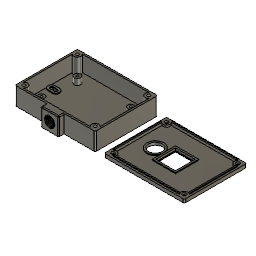
ESP32-FridgeStat Case (Autodesk Fusion 360 design; units mm, degrees)
part number: 2026-06-30-17-07-55-763
Autodesk Fusion 360 part; units mm, degrees
note: some values were not read from the file. Chosen so that the rebuilt part matches the saved one: which bodies a step acts on; which face or edge a step refers to; how an offset face is resized. Set by a fixed rule: which sketch regions a step uses.
sketch "Sketch1" plane through (0, 0, 0) normal (0, 0, 1) x (1, 0, 0)
  line L0 (0, 0) -> (90, 0)
  line L1 (90, 0) -> (90, 70)
  line L2 (90, 70) -> (0, 70)
  line L3 (0, 70) -> (0, 0)
  line L4 (99.999, 69.9991) -> (189.999, 69.9991)
  line L5 (189.999, 69.9991) -> (189.999, -0.0009)
  line L6 (189.999, -0.0009) -> (99.999, -0.0009)
  line L7 (99.999, -0.0009) -> (99.999, 69.9991)
  dimension "d1" = 90
  dimension "d2" = 70
  dimension "d126" = 90
  dimension "d127" = 70
  constraint horizontal L0
  constraint vertical L1
  constraint horizontal L2
  constraint vertical L3
  constraint coincident L0.start L3.end
  constraint horizontal L4
  constraint vertical L5
  constraint horizontal L6
  constraint vertical L7
  measures "d1" distance of L0.start L0.end
  measures "d2" distance of L0.start L2.end
  measures "d126" distance of L4.start L4.end
  measures "d127" distance of L4.start L6.end
extrude "Extrude1" add sketch "Sketch1" along normal blind 2 makes body 1 at (30, 46.6667, 0) makes body 2 at (129.999, 46.6657, 0)
sketch "Sketch3" plane through (0, 0, 2) normal (0, 0, 1) x (-1, 0, 0)
  line L0 (0, -70) -> (0, 0)
  line L1 (0, 0) -> (-90, 0)
  line L2 (-90, 0) -> (-90, -70)
  line L3 (-90, -70) -> (0, -70)
  line L4 (-2, -68) -> (-88, -68)
  line L5 (-88, -68) -> (-88, -2)
  line L6 (-88, -2) -> (-2, -2)
  line L7 (-2, -2) -> (-2, -68)
  circle A0 centre (-5, -65) radius 4
  circle A1 centre (-85, -65) radius 4
  circle A2 centre (-5, -5) radius 4
  circle A3 centre (-85, -5) radius 4
  circle A4 centre (-5, -65) radius 2
  circle A5 centre (-5, -5) radius 2
  circle A6 centre (-85, -65) radius 2
  circle A7 centre (-85, -5) radius 2
  line L8 (0, -70) -> (0, 0)
  line L9 (-90, 0) -> (-90, -70)
  dimension "d23" = 2
  dimension "d24" = 2
  dimension "d25" = 2
  dimension "d26" = 2
  dimension "d27" = 8
  dimension "d28" = 8
  dimension "d29" = 8
  dimension "d30" = 8
  dimension "d31" = 5
  dimension "d32" = 5
  dimension "d33" = 5
  dimension "d34" = 5
  dimension "d35" = 5
  dimension "d36" = 5
  dimension "d37" = 5
  dimension "d38" = 5
  dimension "d39" = 4
  dimension "d40" = 4
  dimension "d41" = 4
  dimension "d42" = 4
  constraint horizontal L4
  constraint vertical L5
  constraint horizontal L6
  constraint vertical L7
  constraint concentric A0 A4
  constraint concentric A2 A5
  constraint concentric A1 A6
  constraint concentric A3 A7
  measures "d23" distance of L0 L7
  measures "d24" distance of L2 L5
  measures "d25" distance of L3 L4
  measures "d26" distance of L1 L6
  measures "d27" diameter of A0
  measures "d28" diameter of A1
  measures "d29" diameter of A2
  measures "d30" diameter of A3
  measures "d31" distance of L0 A0.centre
  measures "d32" distance of L3 A0.centre
  measures "d33" distance of L2 A1.centre
  measures "d34" distance of L3 A1.centre
  measures "d35" distance of L0 A2.centre
  measures "d36" distance of L1 A2.centre
  measures "d37" distance of L2 A3.centre
  measures "d38" distance of L1 A3.centre
  measures "d39" diameter of A4
  measures "d40" diameter of A5
  measures "d41" diameter of A6
  measures "d42" diameter of A7
extrude "Extrude3" add sketch "Sketch3" along normal blind 18 contours L0 L1 L2 L3 L8 L9 | L4 L7 A0 | L4 A0 | L4 L7 A0 | L7 A0 | L4 A1 | L4 L5 A1 | L6 L7 A2 | L7 A2 | L4 L5 A1 | L6 L7 A2 | L6 A2 | L5 A1 | L5 L6 A3 | L6 A3 | L5 A3 | L5 L6 A3 bodies 1
sketch "Sketch7" plane through (0, 0, 0) normal (0, -1, 0) x (1, 0, 0)
  line L0 (0, 0) -> (90, 0)
  line L1 (90, 0) -> (90, 20)
  line L2 (90, 20) -> (0, 20)
  line L3 (0, 20) -> (0, 0)
  line L4 (35, 20) -> (55, 20)
  line L5 (55, 20) -> (55, 0)
  line L6 (55, 0) -> (35, 0)
  line L7 (35, 0) -> (35, 20)
  dimension "d108" = 35
  dimension "d109" = 35
  constraint horizontal L4
  constraint vertical L5
  constraint horizontal L6
  constraint vertical L7
  constraint coincident L0 L5.end
  constraint coincident L2 L4.start
  measures "d108" distance of L3 L7
  measures "d109" distance of L1 L5
extrude "Extrude9" add sketch "Sketch7" along normal blind 6 contours L0 L2 L4 L5 L6 L7 bodies 1
thread "Thread1" "ISO Metric profile 4.0 M4x0.7 M4x0.7 6H" major diameter 4.1095 minor diameter 3.332 pitch 0.7 angle 60 resizes the face on face at (86.3965, 3.5683, 14) on face at (86.843, 65.7769, 14) on face at (3.0025, 5.0997, 14) on face at (6.843, 65.7769, 14) on bodies 1
sketch "Sketch2" plane through (0, 0, 2) normal (0, 0, 1) x (-1, 0, 0)
  circle A0 centre (-15, -15) radius 3.5
  circle A1 centre (-15, -55) radius 3.5
  circle A2 centre (-75, -55) radius 3.5
  circle A3 centre (-75, -15) radius 3.5
  circle A4 centre (-15, -15) radius 1.5
  circle A5 centre (-15, -55) radius 1.5
  circle A6 centre (-75, -55) radius 1.5
  circle A7 centre (-75, -15) radius 1.5
  arc A8 (-7.6458, -2) -> (-2, -7.6458) centre (-5, -5) ccw
  line L0 (-7.6458, -2) -> (-82.3542, -2)
  arc A9 (-88, -7.6458) -> (-82.3542, -2) centre (-85, -5) ccw
  line L1 (-88, -7.6458) -> (-88, -62.3542)
  arc A10 (-82.3542, -68) -> (-88, -62.3542) centre (-85, -65) ccw
  line L2 (-82.3542, -68) -> (-7.6458, -68)
  arc A11 (-2, -62.3542) -> (-7.6458, -68) centre (-5, -65) ccw
  line L3 (-2, -62.3542) -> (-2, -7.6458)
  line L4 (-99.999, 0.0009) -> (-189.999, 0.0009)
  line L5 (-189.999, 0.0009) -> (-189.999, -69.9991)
  line L6 (-189.999, -69.9991) -> (-99.999, -69.9991)
  line L7 (-99.999, -69.9991) -> (-99.999, 0.0009)
  line L8 (0, 0) -> (-35, 0)
  line L9 (-55, 0) -> (-90, 0)
  line L10 (0, -70) -> (0, 0)
  circle A12 centre (-85, -5) radius 1.666
  circle A13 centre (-85, -65) radius 1.666
  circle A14 centre (-5, -5) radius 1.666
  circle A15 centre (-5, -65) radius 1.666
  dimension "d5" = 7
  dimension "d6" = 7
  dimension "d7" = 7
  dimension "d8" = 7
  dimension "d12" = 60
  dimension "d14" = 40
  dimension "d15" = 40
  dimension "d16" = 60
  dimension "d17" = 3
  dimension "d18" = 3
  dimension "d19" = 3
  dimension "d20" = 3
  dimension "d220" = 15
  dimension "d221" = 15
  dimension "d222" = 15
  dimension "d223" = 15
  constraint concentric A0 A4
  constraint concentric A1 A5
  constraint concentric A2 A6
  constraint concentric A3 A7
  measures "d5" diameter of A0
  measures "d6" diameter of A1
  measures "d7" diameter of A2
  measures "d8" diameter of A3
  measures "d12" distance of A0.centre A3.centre
  measures "d14" distance of A0.centre A1.centre
  measures "d15" vertical distance of A2.centre A3.centre
  measures "d16" distance of A1.centre A2.centre
  measures "d17" diameter of A4
  measures "d18" diameter of A5
  measures "d19" diameter of A6
  measures "d20" diameter of A7
  measures "d220" distance of A0.centre L8
  measures "d221" distance of A3.centre L9
  measures "d222" distance of A0.centre L10
  measures "d223" distance of A1.centre L10
extrude "Extrude2" add sketch "Sketch2" along normal blind 7 contours A0 | A1 | A2 | A3 bodies 1
thread "Thread2" "ISO Metric profile 3.0 M3x0.5 M3x0.5 6H" major diameter 3.086 minor diameter 2.529 pitch 0.5 angle 60 resizes the face on face at (74.5223, 13.5781, 6.6667) on face at (73.6827, 54.2826, 4.3333) on face at (13.6827, 54.2826, 4.3333) on face at (13.5075, 15.1494, 6.6667) on bodies 1
sketch "Sketch4" plane through (0, 0, 2) normal (0, 0, 1) x (-1, 0, 0)
  arc A0 (-7.6458, -2) -> (-2, -7.6458) centre (-5, -5) ccw
  line L0 (-7.6458, -2) -> (-82.3542, -2)
  arc A1 (-88, -7.6458) -> (-82.3542, -2) centre (-85, -5) ccw
  line L1 (-88, -7.6458) -> (-88, -62.3542)
  arc A2 (-82.3542, -68) -> (-88, -62.3542) centre (-85, -65) ccw
  line L2 (-82.3542, -68) -> (-7.6458, -68)
  arc A3 (-2, -62.3542) -> (-7.6458, -68) centre (-5, -65) ccw
  line L3 (-2, -62.3542) -> (-2, -7.6458)
  circle A4 centre (-75, -15) radius 3.5
  circle A5 centre (-75, -55) radius 3.5
  circle A6 centre (-15, -55) radius 3.5
  circle A7 centre (-15, -15) radius 3.5
  circle A8 centre (-11, -35) radius 4
  circle A9 centre (-6, -35) radius 4
  circle A10 centre (-84, -37.5) radius 4
  circle A11 centre (-84, -32.5) radius 4
  line L4 (0, -70) -> (0, 0)
  line L5 (-90, -70) -> (0, -70)
  line L6 (-90, 0) -> (-90, -70)
  circle A12 centre (-6, -35) radius 1.75
  circle A13 centre (-84, -37.5) radius 1.75
  circle A14 centre (-11, -35) radius 1.75
  circle A15 centre (-84, -32.5) radius 1.75
  line L7 (0, 0) -> (-35, 0)
  line L8 (-55, 0) -> (-90, 0)
  line L9 (-90, -70) -> (0, -70)
  line L10 (-11, -39) -> (-6, -39)
  line L11 (-6, -39) -> (-6, -31)
  line L12 (-6, -31) -> (-11, -31)
  line L13 (-11, -31) -> (-11, -39)
  line L14 (-80, -37.5) -> (-88, -37.5)
  line L15 (-88, -37.5) -> (-88, -32.5)
  line L16 (-88, -32.5) -> (-80, -32.5)
  line L17 (-80, -32.5) -> (-80, -37.5)
  line L18 (-6, -36.75) -> (-11, -36.75)
  line L19 (-11, -36.75) -> (-11, -33.25)
  line L20 (-11, -33.25) -> (-6, -33.25)
  line L21 (-6, -33.25) -> (-6, -36.75)
  line L22 (-82.25, -37.5) -> (-85.75, -37.5)
  line L23 (-85.75, -37.5) -> (-85.75, -32.5)
  line L24 (-85.75, -32.5) -> (-82.25, -32.5)
  line L25 (-82.25, -32.5) -> (-82.25, -37.5)
  dimension "d55" = 8
  dimension "d56" = 8
  dimension "d57" = 8
  dimension "d58" = 8
  dimension "d61" = 35
  dimension "d62" = 6
  dimension "d63" = 6
  dimension "d64" = 32.5
  dimension "d65" = 6
  dimension "d67" = 3.5
  dimension "d68" = 3.5
  dimension "d69" = 3.5
  dimension "d70" = 3.5
  dimension "d123" = 5
  dimension "d124" = 35
  dimension "d125" = 5
  constraint concentric A9 A12
  constraint concentric A10 A13
  constraint concentric A8 A14
  constraint concentric A11 A15
  constraint horizontal L10
  constraint vertical L11
  constraint horizontal L12
  constraint vertical L13
  constraint coincident A9 L11.end
  constraint coincident A8 L10.start
  constraint horizontal L14
  constraint vertical L15
  constraint horizontal L16
  constraint vertical L17
  constraint coincident A11 L15.end
  constraint coincident A10 L14.start
  constraint horizontal L18
  constraint vertical L19
  constraint horizontal L20
  constraint vertical L21
  constraint coincident A14 L19.end
  constraint coincident L13 L19.end
  constraint coincident L11 L18.start
  constraint coincident A12 L18.start
  constraint horizontal L22
  constraint vertical L23
  constraint horizontal L24
  constraint vertical L25
  constraint coincident L16 L23.end
  constraint coincident A15 L23.end
  constraint coincident L14 L22.start
  constraint coincident A13 L22.start
  measures "d55" diameter of A8
  measures "d56" diameter of A9
  measures "d57" diameter of A10
  measures "d58" diameter of A11
  measures "d61" distance of A9.centre L5
  measures "d62" distance of A9.centre L4
  measures "d63" distance of A10.centre L6
  measures "d64" distance of A10.centre L5
  measures "d65" distance of A11.centre L6
  measures "d67" diameter of A12
  measures "d68" diameter of A13
  measures "d69" diameter of A14
  measures "d70" diameter of A15
  measures "d123" distance of A10.centre A11.centre
  measures "d124" distance of A8.centre L9
  measures "d125" distance of A8.centre A9.centre
extrude "Extrude5" cut sketch "Sketch4" against normal up to surface (2 mm away) contours A8 A12 L11 L21 | A12 L11 L21 | A8 A12 L20 | A8 A12 L18 | A10 A15 L16 L24 | A15 L16 L24 | A10 A15 L23 | A8 A9 A12 A14 L18 L20 | A9 A14 L20 | A8 A12 | A14 L13 L19 | A9 A14 L13 L19 | A9 A14 L18 | A13 L14 L22 | A11 A13 L23 | A11 A13 L14 L22 | A10 A15 L25 | A10 A11 A13 A15 L23 L25 | A10 A15 | A9 A14 | A11 A13 L25 | A11 A13 bodies 1
extrude "Extrude6" add sketch "Sketch4" along normal blind 1 separate body contours A9 A12 L11 | A8 A9 L11 L20 | A8 A9 L12 | A8 A9 L10 | A8 A9 L11 L18 | L1 A10 A11 L15 | A10 A11 L16 L23 | A11 A15 L16 | A8 A9 L13 L20 | A8 A9 L20 | A8 A14 L13 | A8 A9 L18 | A8 A9 L13 L18 | A10 A13 L14 | A10 A11 L14 L23 | A10 A11 L17 | A10 A11 L16 L25 | A10 A11 L23 | A10 A11 L14 L25 | A10 A11 L25 makes body 3 at (87.25, 34.1667, 2) makes body 4 at (9.3333, 32.5, 3)
fillet "Fillet3" radius 1.5 4 edges at (90, 0, 10) (90, 70, 10) (0, 0, 10) (0, 70, 10) on bodies 1
fillet "Fillet3" radius 1 5 edges at (35, -6, 10) (45, -6, 20) (55, -6, 10) (55, -3, 20) (35, -3, 20) on bodies 1
sketch "Sketch8" plane through (0, -6, 0) normal (0, -1, 0) x (1, 0, 0)
  line L0 (54, 0) -> (54, 19)
  line L1 (54, 19) -> (36, 19)
  line L2 (36, 19) -> (36, 0)
  line L3 (36, 0) -> (54, 0)
  circle A0 centre (45, 10) radius 6
  line L4 (35, 19) -> (35, 0)
  line L5 (0, 0) -> (90, 0)
  dimension "d116" = 12
  dimension "d117" = 10
  dimension "d118" = 10
  measures "d116" diameter of A0
  measures "d117" distance of A0.centre L4
  measures "d118" distance of A0.centre L5
extrude "Extrude10" cut sketch "Sketch8" against normal up to surface (8 mm away) contours A0 bodies 1
thread "Thread5" "ISO Metric profile 12.0 M12x1.5 M12x1.5 6H" major diameter 12.203 minor diameter 10.526 pitch 1.5 angle 60 modelled right hand crest width 0.4065 on face at (50.9925, -0.6667, 9.7009) crest through (50.263, -5.625, 10) on bodies 1
sketch "Sketch9" plane through (0, 0, 2) normal (0, 0, 1) x (-1, 0, 0)
  line L0 (-99.999, 0.0009) -> (-189.999, 0.0009)
  line L1 (-189.999, 0.0009) -> (-189.999, -69.9991)
  line L2 (-189.999, -69.9991) -> (-99.999, -69.9991)
  line L3 (-99.999, -69.9991) -> (-99.999, 0.0009)
  line L4 (-103.499, -66.4991) -> (-186.499, -66.4991)
  line L5 (-186.499, -66.4991) -> (-186.499, -3.4991)
  line L6 (-186.499, -3.4991) -> (-103.499, -3.4991)
  line L7 (-103.499, -3.4991) -> (-103.499, -66.4991)
  circle A0 centre (-104.999, -64.9991) radius 4
  circle A1 centre (-184.999, -64.9991) radius 4
  circle A2 centre (-104.999, -4.9991) radius 4
  circle A3 centre (-184.999, -4.9991) radius 4
  line L8 (-134.999, -44.9991) -> (-154.999, -44.9991)
  line L9 (-154.999, -44.9991) -> (-154.999, -24.9991)
  line L10 (-154.999, -24.9991) -> (-134.999, -24.9991)
  line L11 (-134.999, -24.9991) -> (-134.999, -44.9991)
  line L12 (-133.999, -45.9991) -> (-155.999, -45.9991)
  line L13 (-155.999, -45.9991) -> (-155.999, -23.9991)
  line L14 (-155.999, -23.9991) -> (-133.999, -23.9991)
  line L15 (-133.999, -23.9991) -> (-133.999, -45.9991)
  circle A4 centre (-122.499, -34.9991) radius 7.5
  line L16 (-131.999, -47.9991) -> (-157.999, -47.9991)
  line L17 (-157.999, -47.9991) -> (-157.999, -21.9991)
  line L18 (-157.999, -21.9991) -> (-131.999, -21.9991)
  line L19 (-131.999, -21.9991) -> (-131.999, -47.9991)
  circle A5 centre (-122.499, -34.9991) radius 9.5
  dimension "d128" = 3.5
  dimension "d129" = 3.5
  dimension "d130" = 3.5
  dimension "d131" = 3.5
  dimension "d132" = 8
  dimension "d133" = 8
  dimension "d134" = 8
  dimension "d135" = 8
  dimension "d136" = 5
  dimension "d137" = 5
  dimension "d138" = 5
  dimension "d139" = 5
  dimension "d140" = 5
  dimension "d141" = 5
  dimension "d142" = 5
  dimension "d143" = 5
  dimension "d152" = 22
  dimension "d153" = 26
  dimension "d154" = 20
  dimension "d155" = 32
  dimension "d156" = 34
  dimension "d157" = 35
  dimension "d158" = 20
  dimension "d159" = 22
  dimension "d160" = 26
  dimension "d161" = 22
  dimension "d162" = 24
  dimension "d163" = 25
  dimension "d164" = 22.5
  dimension "d165" = 35
  dimension "d204" = 15
  dimension "d242" = 19
  constraint horizontal L4
  constraint vertical L5
  constraint horizontal L6
  constraint vertical L7
  constraint horizontal L8
  constraint vertical L9
  constraint horizontal L10
  constraint vertical L11
  constraint horizontal L12
  constraint vertical L13
  constraint horizontal L14
  constraint vertical L15
  constraint horizontal L16
  constraint vertical L17
  constraint horizontal L18
  constraint vertical L19
  constraint coincident A4.centre A5.centre
  measures "d128" distance of L3 L7
  measures "d129" distance of L2 L4
  measures "d130" distance of L0 L6
  measures "d131" distance of L1 L5
  measures "d132" diameter of A0
  measures "d133" diameter of A1
  measures "d134" diameter of A2
  measures "d135" diameter of A3
  measures "d136" distance of L3 A0.centre
  measures "d137" distance of L2 A0.centre
  measures "d138" distance of L2 A1.centre
  measures "d139" distance of L1 A1.centre
  measures "d140" distance of L3 A2.centre
  measures "d141" distance of L0 A2.centre
  measures "d142" distance of L0 A3.centre
  measures "d143" distance of L1 A3.centre
  measures "d152" distance of L13 L15
  measures "d153" distance of L17 L19
  measures "d154" distance of L9 L11
  measures "d155" distance of L3 L19
  measures "d156" distance of L3 L15
  measures "d157" distance of L3 L11
  measures "d158" distance of L8 L10
  measures "d159" distance of L12 L14
  measures "d160" distance of L16 L18
  measures "d161" distance of L0 L18
  measures "d162" distance of L0 L14
  measures "d163" distance of L0 L10
  measures "d164" distance of L3 A4.centre
  measures "d165" distance of L2 A4.centre
  measures "d204" diameter of A4
  measures "d242" diameter of A5
extrude "Extrude11" add sketch "Sketch9" along normal blind 2 contours L0 L1 L2 L3 | L4 L7 A0 | L4 L7 A0 | L4 L5 A1 | L4 L5 A1 | L6 L7 A2 | L6 L7 A2 | L5 L6 A3 | L5 L6 A3 bodies 2
extrude "Extrude13" cut sketch "Sketch9" against normal up to surface (2 mm away) contours L8 L9 L10 L11 | A4 bodies 2
extrude "Extrude14" cut sketch "Sketch9" against normal blind 1.4 contours L12 L13 L14 L15 bodies 2
extrude "Extrude15" add sketch "Sketch9" along normal blind 1 contours A5 | L16 L17 L18 L19 bodies 2
sketch "Sketch10" plane through (0, 0, 0) normal (0, 0, -1) x (1, 0, 0)
  circle A0 centre (122.499, -34.9991) radius 7.5
  line L0 (134.999, -44.9991) -> (134.999, -24.9991)
  line L1 (134.999, -24.9991) -> (154.999, -24.9991)
  line L2 (154.999, -24.9991) -> (154.999, -44.9991)
  line L3 (154.999, -44.9991) -> (134.999, -44.9991)
  line L4 (189.999, 0.0009) -> (99.999, 0.0009)
  line L5 (99.999, 0.0009) -> (99.999, -69.9991)
  line L6 (99.999, -69.9991) -> (189.999, -69.9991)
  line L7 (189.999, -69.9991) -> (189.999, 0.0009)
  circle A1 centre (104.999, -64.9991) radius 3.75
  circle A2 centre (104.999, -4.9991) radius 3.75
  circle A3 centre (184.999, -4.9991) radius 3.75
  circle A4 centre (184.999, -64.9991) radius 3.75
  dimension "d172" = 7.5
  dimension "d173" = 7.5
  dimension "d174" = 7.5
  dimension "d175" = 7.5
  dimension "d224" = 5
  dimension "d225" = 5
  dimension "d226" = 5
  dimension "d227" = 5
  dimension "d228" = 5
  dimension "d229" = 5
  dimension "d230" = 5
  dimension "d231" = 5
  measures "d172" diameter of A1
  measures "d173" diameter of A2
  measures "d174" diameter of A3
  measures "d175" diameter of A4
  measures "d224" distance of L7 A3.centre
  measures "d225" distance of L4 A3.centre
  measures "d226" distance of L6 A4.centre
  measures "d227" distance of L7 A4.centre
  measures "d228" distance of L6 A1.centre
  measures "d229" distance of L5 A1.centre
  measures "d230" distance of L5 A2.centre
  measures "d231" distance of L4 A2.centre
extrude "Extrude19" cut sketch "Sketch10" against normal blind 0.4 contours A1 | A2 | A3 | A4 bodies 2
sketch "Sketch12" plane through (0, 0, 0) normal (0, 0, -1) x (1, 0, 0)
  circle A0 centre (104.999, -64.9991) radius 2.05
  circle A1 centre (184.999, -64.9991) radius 2.05
  circle A2 centre (184.999, -4.9991) radius 2.05
  circle A3 centre (104.999, -4.9991) radius 2.05
  line L0 (189.999, -69.9991) -> (99.999, -69.9991)
  line L1 (99.999, 0.0009) -> (189.999, 0.0009)
  line L2 (189.999, 0.0009) -> (189.999, -69.9991)
  line L3 (99.999, -69.9991) -> (99.999, 0.0009)
  dimension "d184" = 4.1
  dimension "d185" = 4.1
  dimension "d186" = 4.1
  dimension "d187" = 4.1
  dimension "d232" = 5
  dimension "d233" = 5
  dimension "d234" = 5
  dimension "d235" = 5
  dimension "d236" = 5
  dimension "d237" = 5
  dimension "d238" = 5
  dimension "d239" = 5
  measures "d184" diameter of A0
  measures "d185" diameter of A1
  measures "d186" diameter of A2
  measures "d187" diameter of A3
  measures "d232" distance of A0.centre L0
  measures "d233" distance of A3.centre L1
  measures "d234" distance of A2.centre L2
  measures "d235" distance of A2.centre L1
  measures "d236" distance of A1.centre L0
  measures "d237" distance of A1.centre L2
  measures "d238" distance of A0.centre L3
  measures "d239" distance of A3.centre L3
extrude "Extrude20" cut sketch "Sketch12" against normal up to surface (4 mm away) contours A0 | A1 | A2 | A3 bodies 2
extrude "Extrude21" cut sketch "Sketch10" against normal blind 1.8 draft -45 from surface at -0.4 contours A1 bodies 2
extrude "Extrude22" cut sketch "Sketch10" against normal blind 1.8 draft -45 from surface at -0.4 contours A4 bodies 2
extrude "Extrude23" cut sketch "Sketch10" against normal blind 1.8 draft -45 from surface at -0.4 contours A3 bodies 2
extrude "Extrude24" cut sketch "Sketch10" against normal blind 1.8 draft -45 from surface at -0.4 contours A2 bodies 2
fillet "Fillet4" radius 1.5 4 edges at (189.999, -0.0009, 2) (189.999, 69.9991, 2) (99.999, 69.9991, 2) (99.999, -0.0009, 2) on bodies 2
sketch "Sketch13" plane through (0, 0, 4) normal (0, 0, 1) x (-1, 0, 0)
  arc A0 (-99.999, -1.4991) -> (-101.499, 0.0009) centre (-101.499, -1.4991) ccw
  line L0 (-101.499, 0.0009) -> (-188.499, 0.0009)
  arc A1 (-188.499, 0.0009) -> (-189.999, -1.4991) centre (-188.499, -1.4991) ccw
  line L1 (-189.999, -1.4991) -> (-189.999, -68.4991)
  arc A2 (-189.999, -68.4991) -> (-188.499, -69.9991) centre (-188.499, -68.4991) ccw
  line L2 (-188.499, -69.9991) -> (-101.499, -69.9991)
  arc A3 (-101.499, -69.9991) -> (-99.999, -68.4991) centre (-101.499, -68.4991) ccw
  line L3 (-99.999, -68.4991) -> (-99.999, -1.4991)
  line L4 (-186.499, -61.291) -> (-186.499, -8.7072)
  arc A4 (-186.499, -8.7072) -> (-181.2909, -3.4991) centre (-184.999, -4.9991) ccw
  line L5 (-181.2909, -3.4991) -> (-108.7071, -3.4991)
  arc A5 (-108.7071, -3.4991) -> (-103.499, -8.7072) centre (-104.999, -4.9991) ccw
  line L6 (-103.499, -8.7072) -> (-103.499, -61.291)
  arc A6 (-103.499, -61.291) -> (-108.7071, -66.4991) centre (-104.999, -64.9991) ccw
  line L7 (-108.7071, -66.4991) -> (-181.2909, -66.4991)
  arc A7 (-181.2909, -66.4991) -> (-186.499, -61.291) centre (-184.999, -64.9991) ccw
  line L8 (-102.099, -67.8991) -> (-187.899, -67.8991)
  line L9 (-187.899, -67.8991) -> (-187.899, -2.0991)
  line L10 (-187.899, -2.0991) -> (-102.099, -2.0991)
  line L11 (-102.099, -2.0991) -> (-102.099, -67.8991)
  circle A8 centre (-184.999, -64.9991) radius 4.1
  circle A9 centre (-184.999, -64.9991) radius 4.1
  circle A10 centre (-104.999, -4.9991) radius 4.1
  circle A11 centre (-104.999, -4.9991) radius 4.1
  circle A12 centre (-184.999, -4.9991) radius 2.05
  circle A13 centre (-104.999, -4.9991) radius 2.05
  circle A14 centre (-184.999, -64.9991) radius 2.05
  circle A15 centre (-104.999, -64.9991) radius 2.05
  circle A16 centre (-104.999, -64.9991) radius 4.1
  circle A17 centre (-184.999, -4.9991) radius 4.1
  point P0 (-185.999, -3.9991)
  point P1 (-103.999, -3.9991)
  point P2 (-185.999, -65.9991)
  point P3 (-103.999, -65.9991)
  point P4 (-185.999, -3.9991)
  point P5 (-103.999, -3.9991)
  point P6 (-185.999, -65.9991)
  point P7 (-103.999, -65.9991)
  dimension "d210" = 2.1
  dimension "d211" = 2.1
  dimension "d212" = 2.1
  dimension "d213" = 2.1
  dimension "d214" = 8.2
  dimension "d215" = 8.2
  dimension "d216" = 8.2
  dimension "d217" = 8.2
  dimension "d240" = 8.2
  dimension "d241" = 8.2
  constraint horizontal L8
  constraint vertical L9
  constraint horizontal L10
  constraint vertical L11
  constraint concentric A8 A14
  constraint concentric A10 A13
  constraint coincident A5.centre A10.centre
  constraint coincident A7.centre A8.centre
  constraint coincident A6.centre A15.centre
  constraint coincident A4.centre A12.centre
  measures "d210" distance of L3 L11
  measures "d211" distance of L1 L9
  measures "d212" distance of L2 L8
  measures "d213" distance of L0 L10
  measures "d214" diameter of A8
  measures "d215" diameter of A9
  measures "d216" diameter of A10
  measures "d217" diameter of A11
  measures "d240" diameter of A16
  measures "d241" diameter of A17
extrude "Extrude26" add sketch "Sketch13" along normal blind 1 contours L4 L9 A8 A9 A17 | L7 L8 A8 A9 A16 | L5 L10 A10 A11 A17 | L6 L11 A10 A11 A16 bodies 2
